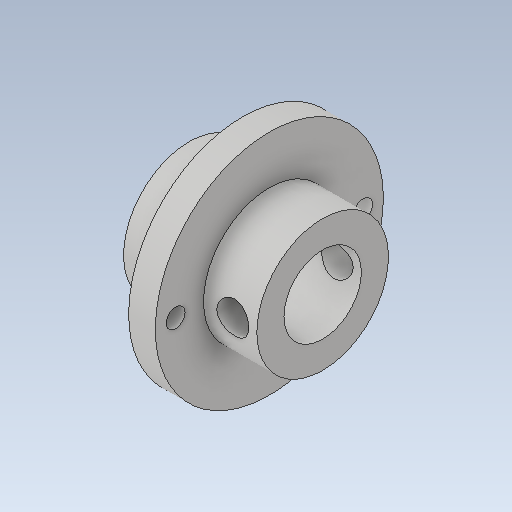
# Autodesk Inventor part: Переходник Чугун СЧ15
Saved by Autodesk Inventor 2020 (Build 240168000, 168)
## iProperties
Created: 2019-04-05
Part Number: Переходник Чугун СЧ15
Material: Типовые
Document SubType Name: Modeling
Designer: гей
Density: 1 g/cm^3
Appearance: По умолчанию
Author: гей
Autodesk Inventor part; units mm, degrees
ref_plane "YZ Plane" through (0, 0, 0) normal (1, 0, 0) x (0, 1, 0)
ref_plane "XZ Plane" through (0, 0, 0) normal (0, 1, 0) x (-1, 0, 0)
ref_plane "XY Plane" through (0, 0, 0) normal (0, 0, 1) x (1, 0, 0)
sketch "Эскиз1" plane through (0, 0, 0) normal (1, 0, 0) x (0, 1, 0)
  circle A0 centre (0, 0) radius 132.5
  dimension "d0" = 265
  constraints: 1 centre point, 1 coincident
  measures "d0" diameter of A0
extrude "Выдавливание1" add sketch "Эскиз1" along normal mid plane 31
sketch "Эскиз2" plane through (15.5, 0, 0) normal (1, 0, 0) x (0, 0, -1)
  circle A0 centre (0, 0) radius 76.5
  dimension "d3" = 153
  constraints: 1 centre point, 1 coincident
  measures "d3" diameter of A0
extrude "Выдавливание2" add sketch "Эскиз2" along normal blind 62
sketch "Эскиз3" plane through (-15.5, 0, 0) normal (-1, 0, 0) x (0, 0, 1)
  circle A0 centre (0, 0) radius 76.5
  dimension "d6" = 153
  constraints: 1 centre point, 1 coincident
  measures "d6" diameter of A0
extrude "Выдавливание3" add sketch "Эскиз3" along normal blind 62
sketch "Эскиз4" plane through (-77.5, 0, 0) normal (-1, 0, 0) x (0, 0, 1)
  circle A0 centre (0, 0) radius 45
  dimension "d9" = 90
  constraints: 1 centre point, 1 coincident
  measures "d9" diameter of A0
extrude "Выдавливание4" cut sketch "Эскиз4" against normal through all
sketch "Эскиз5" plane through (0, 0, 0) normal (0, 0, 1) x (1, 0, 0)
  circle A0 centre (49.5, 0) radius 18.5
  line L0 (77.5, 45) -> (77.5, -45) projected
  point P0 (0, 0)
  dimension "d12" = 28
  dimension "d13" = 37
  constraints: 1 centre point
  measures "d12" distance from line of L0 A0.centre
  measures "d13" diameter of A0
extrude "Выдавливание5" cut sketch "Эскиз5" along normal through all both and the other way through all
sketch "Эскиз7" plane through (15.5, 0, 0) normal (1, 0, 0) x (0, 0, -1)
  circle A0 centre (-109, 0) radius 11
  circle A1 centre (109, 0) radius 11
  point P0 (0, 0)
  dimension "d16" = 109
  dimension "d17" = 109
  dimension "d18" = 22
  dimension "d19" = 22
  constraints: 2 centre point
  measures "d16" distance of point (0, 0) A0.centre
  measures "d17" distance of A1.centre point (0, 0)
  measures "d18" diameter of A0
  measures "d19" diameter of A1
extrude "Выдавливание6" cut sketch "Эскиз7" against normal through all
sketch "Эскиз8" plane through (0, 0, 0) normal (0, 1, 0) x (-1, 0, 0)
  point P0 (0, 0)
